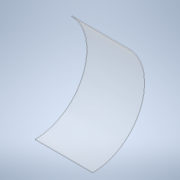
# Autodesk Inventor part: Lexan Glock Back
Saved by Autodesk Inventor 2021 (Build 250183000, 183)
## iProperties
Created: 2021-02-04
Part Number: Lexan Glock Back
Material: Polycarbonate, Clear
Document SubType Name: Modeling
Designer: aidan
Density: 1.2 g/cm^3
Appearance: Polycarbonate - Clear
Author: aidan
Autodesk Inventor part; units mm, degrees
ref_plane "YZ Plane" through (0, 0, 0) normal (1, 0, 0) x (0, 1, 0)
ref_plane "XZ Plane" through (0, 0, 0) normal (0, 1, 0) x (-1, 0, 0)
ref_plane "XY Plane" through (0, 0, 0) normal (0, 0, 1) x (1, 0, 0)
sketch "Sketch1" plane through (0, 0, 0) normal (1, 0, 0) x (0, 1, 0)
  arc A0 (-209.55, 0) -> (148.1742, -148.1742) centre (0, 0) ccw
  line L0 (-209.55, 0) -> (0, 0) construction
  line L1 (0, 0) -> (148.1742, -148.1742) construction
  arc A1 (-212.5472, 0) -> (150.2936, -150.2936) centre (0, 0) ccw
  line L2 (-212.5261, 2.9972) -> (1.2415, 2.9972) construction
  line L3 (1.2415, 2.9972) -> (152.398, -148.1593) construction
  line L4 (148.1742, -148.1742) -> (150.2936, -150.2936)
  line L5 (-209.55, 0) -> (-212.5472, 0)
  dimension "d0" = 209.55
  dimension "d1" = 2.9972
  dimension "d2" = 135
  constraints: 12 end point, 4 point on circle, 2 centre point, 2 collinear, 1 coincident, 1 horizontal, 1 other
  measures "d0" radius of A0
  measures "d1" radial gap between concentric circles of A0 A1
  measures "d2" angle of L1 L0
extrude "Extrusion1" add sketch "Sketch1" along normal blind 234.95
body "Solid1"
